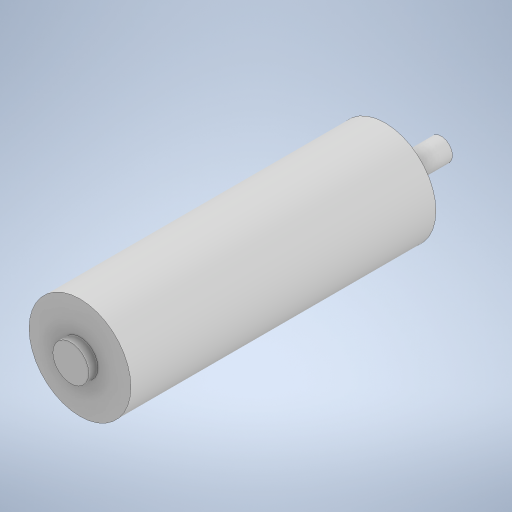
# Autodesk Inventor part: DriveMotor
Saved by Autodesk Inventor 2024 (Build 280153000, 153)
## iProperties
Created: 2025-01-04
Part Number: DriveMotor
Material: Generic
Document SubType Name: Modeling
Designer: Tommy Rohmann
Density: 1 g/cm^3
Appearance: Default
Author: Tommy Rohmann
Autodesk Inventor part; units mm, degrees
ref_plane "YZ Plane" through (0, 0, 0) normal (1, 0, 0) x (0, 1, 0)
ref_plane "XZ Plane" through (0, 0, 0) normal (0, 1, 0) x (-1, 0, 0)
ref_plane "XY Plane" through (0, 0, 0) normal (0, 0, 1) x (1, 0, 0)
sketch "Sketch1" plane through (0, 0, 0) normal (0, 0, 1) x (1, 0, 0)
  circle A0 centre (0, 0) radius 18.0213
  circle A1 centre (0, 0) radius 4
  circle A2 centre (0, 0) radius 11.0236
  circle A3 centre (0, 0) radius 6.35
  dimension "d0" = 36.0426
  dimension "d1" = 8
  dimension "d2" = 22.0472
  dimension "d9" = 12.7
  constraints: 4 centre point, 4 coincident
  measures "d0" diameter of A0
  measures "d1" diameter of A1
  measures "d2" diameter of A2
  measures "d9" diameter of A3
extrude "Extrusion1" add sketch "Sketch1" along normal blind 107.95 contours A0 | A1 | A2 | A3
extrude "Extrusion2" add sketch "Sketch1" against normal blind 2.0701 contours A2 | A3
extrude "Extrusion3" add sketch "Sketch1" against normal blind 19.9009 contours A1
extrude "Extrusion4" add sketch "Sketch1" along normal blind 111.2012 contours A1 | A3
body "Solid1"
